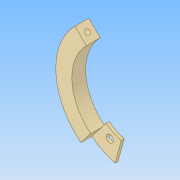
# Autodesk Inventor part: BearingMount1
Saved by Autodesk Inventor 2017.3 (Build 213256000, 256)
## iProperties
Created: 2019-06-26
Part Number: BearingMount1
Material: ABS Plastic
Document SubType Name: Modeling
Designer: Derek Wider
Density: 1.06 g/cm^3
Appearance: Beige
Author: Derek Wider
Autodesk Inventor part; units mm, degrees
ref_plane "YZ Plane" through (0, 0, 0) normal (1, 0, 0) x (0, 1, 0)
ref_plane "XZ Plane" through (0, 0, 0) normal (0, 1, 0) x (-1, 0, 0)
ref_plane "XY Plane" through (0, 0, 0) normal (0, 0, 1) x (1, 0, 0)
sketch "Sketch1" plane through (0, 0, 0) normal (0, 0, 1) x (1, 0, 0)
  circle A0 centre (0, 0) radius 25.4
  circle A1 centre (0, 0) radius 33.655
  line L0 (-17.9605, 17.9605) -> (-23.7977, 23.7977)
  line L1 (17.9605, 17.9605) -> (23.7977, 23.7977)
  line L2 (-23.7977, 23.7977) -> (-23.7977, 0) construction
  line L3 (23.7977, 23.7977) -> (23.7977, 0) construction
  line L4 (-6.574, -24.5345) -> (-8.7106, -32.5082)
  line L5 (6.574, -24.5345) -> (8.7106, -32.5082)
  line L6 (-6.574, -24.5345) -> (-6.574, 0) construction
  line L7 (6.574, -24.5345) -> (6.574, 0) construction
  dimension "d0" = 50.8
  dimension "d1" = 67.31
  dimension "d2" = 90
  dimension "d3" = 30
  constraints: 16 end point, 8 point on circle, 4 horizontal alignment, 4 line through centre, 4 vertical, 2 centre point, 2 coincident, 2 parallel
  measures "d0" diameter of A0
  measures "d1" diameter of A1
extrude "Extrusion1" add sketch "Sketch1" along normal blind 7.112 contours A0 L4 A1 L0
sketch "Sketch2" plane through (-23.7977, 23.7977, 0) normal (0.7071068, 0.7071068, 0) x (-0.7071068, 0.7071068, 0)
  line L0 (-8.255, 0) -> (0, 0) construction
  line L1 (0, 0) -> (0, 7.112) construction
  line L2 (-8.255, 7.112) -> (0, 7.112) construction
  line L3 (-8.255, 0) -> (-8.255, 7.112) construction
  circle A0 centre (-4.1275, 3.556) radius 1.27
  point P0 (-33.655, 0)
  dimension "d6" = 2.54
  constraints: 1 centre point
  measures "d6" diameter of A0
extrude "Extrusion2" cut sketch "Sketch2" against normal blind 10.16
sketch "Sketch3" plane through (0, 0, 7.112) normal (0, 0, 1) x (1, 0, 0)
  line L0 (-17.9605, 17.9605) -> (-23.7977, 23.7977) projected
  arc A0 (-23.7977, 23.7977) -> (-8.7106, -32.5082) centre (0, 0) ccw projected
  line L1 (-8.7106, -32.5082) -> (-6.574, -24.5345) projected
  arc A1 (-17.9605, 17.9605) -> (-6.574, -24.5345) centre (0, 0) ccw projected
  line L2 (-15.6378, -20.0155) -> (-20.7201, -26.5205)
  dimension "d9" = 23
  constraints: 2 end point, 2 point on circle, 1 line through centre
extrude "Extrusion3" cut sketch "Sketch3" against normal blind 5.588 contours A1 L1 A0 L2
sketch "Sketch5" plane through (0, 0, 1.524) normal (0, 0, 1) x (1, 0, 0)
  line L0 (-6.574, -24.5345) -> (-8.7106, -32.5082) projected
  arc A0 (-15.6378, -20.0155) -> (-6.574, -24.5345) centre (0, 0) ccw projected
  line L1 (-20.7201, -26.5205) -> (-15.6378, -20.0155) projected
  arc A1 (-20.7201, -26.5205) -> (-8.7106, -32.5082) centre (0, 0) ccw projected
  line L2 (-6.574, -24.5345) -> (-5.5879, -20.8543)
  line L3 (-15.6378, -20.0155) -> (-13.2921, -17.0132)
  arc A2 (-13.2921, -17.0132) -> (-5.5879, -20.8543) centre (0, 0) ccw
  line L4 (-6.574, -24.5345) -> (-8.7106, -32.5082) projected
  line L5 (-20.7201, -26.5205) -> (-15.6378, -20.0155) projected
  dimension "d18" = 3.81
  constraints: 4 end point, 2 collinear, 2 point on circle, 1 centre point, 1 coincident
  measures "d18" distance of L0.start L2.end
extrude "Extrusion5" add sketch "Sketch5" against normal up to surface (1.524 mm away)
sketch "Sketch6" plane through (0, 0, 1.524) normal (0, 0, 1) x (1, 0, 0)
  circle A0 centre (-11.4468, -22.9586) radius 1.905
  line L0 (0, 0) -> (0, -28.075) construction
  dimension "d21" = 3.81
  dimension "d22" = 25.654
  dimension "d23" = 26.5
  constraints: 2 end point, 1 centre point, 1 vertical
  measures "d21" diameter of A0
  measures "d22" distance of A0.centre L0.start
extrude "Extrusion6" cut sketch "Sketch6" against normal blind 25.4
body "Solid1"
